Autodesk Inventor part; units mm, degrees
(part 2 of 2)
  spline S182 degree 2 poles (-123.4391, 76.8536) (-123.4391, 75.1966) (-121.7718, 73.4367) (-120.2898, 73.4367) knots 0 0 0 1 2 2 2
  spline S183 degree 2 poles (-120.2898, 73.4367) (-119.7649, 73.4367) (-118.746, 73.6734) (-118.3344, 73.8587) knots 0 0 0 1 2 2 2
  spline S184 degree 2 poles (-118.3344, 73.8587) (-117.9021, 74.0645) (-117.3052, 74.4247) (-117.1096, 74.5894) knots 0 0 0 1 2 2 2
  line L455 (-117.1096, 74.5894) -> (-117.017, 74.5894)
  line L456 (-117.017, 74.5894) -> (-117.017, 72.8398)
  spline S185 degree 2 poles (-117.017, 72.8398) (-117.2949, 72.7266) (-118.1388, 72.3972) (-118.4682, 72.3046) knots 0 0 0 1 2 2 2
  spline S186 degree 2 poles (-118.4682, 72.3046) (-118.9313, 72.1708) (-119.6929, 72.037) (-120.2692, 72.037) knots 0 0 0 1 2 2 2
  spline S187 degree 2 poles (-118.4064, 78.0783) (-118.427, 78.7267) (-118.6946, 79.6735) (-118.9519, 79.9925) knots 0 0 0 1 2 2 2
  spline S188 degree 2 poles (-118.9519, 79.9925) (-119.2297, 80.3527) (-120.1045, 80.7335) (-120.7529, 80.7335) knots 0 0 0 1 2 2 2
  spline S189 degree 2 poles (-120.7529, 80.7335) (-121.391, 80.7335) (-122.2864, 80.3527) (-122.6569, 79.9822) knots 0 0 0 1 2 2 2
  spline S190 degree 2 poles (-122.6569, 79.9822) (-123.0171, 79.6014) (-123.3876, 78.6855) (-123.4391, 78.0783) knots 0 0 0 1 2 2 2
  line L457 (-123.4391, 78.0783) -> (-118.4064, 78.0783)
  line L458 (-107.8162, 72.2532) -> (-109.7819, 72.2532)
  line L459 (-109.7819, 72.2532) -> (-112.0976, 75.8347)
  line L460 (-112.0976, 75.8347) -> (-114.475, 72.2532)
  line L461 (-114.475, 72.2532) -> (-116.2966, 72.2532)
  line L462 (-116.2966, 72.2532) -> (-112.993, 76.9771)
  line L463 (-112.993, 76.9771) -> (-116.2657, 81.7833)
  line L464 (-116.2657, 81.7833) -> (-114.3, 81.7833)
  line L465 (-114.3, 81.7833) -> (-111.9947, 78.2326)
  line L466 (-111.9947, 78.2326) -> (-109.6378, 81.7833)
  line L467 (-109.6378, 81.7833) -> (-107.8162, 81.7833)
  line L468 (-107.8162, 81.7833) -> (-111.0993, 77.08)
  line L469 (-111.0993, 77.08) -> (-107.8162, 72.2532)
  spline S191 degree 2 poles (-101.2604, 73.2617) (-101.4559, 73.1177) (-102.1146, 72.6031) (-102.4233, 72.4487) knots 0 0 0 1 2 2 2
  spline S192 degree 2 poles (-102.4233, 72.4487) (-102.8453, 72.2223) (-103.6378, 71.9856) (-104.3582, 71.9856) knots 0 0 0 1 2 2 2
  spline S193 degree 2 poles (-104.3582, 71.9856) (-104.9448, 71.9856) (-106.0049, 72.4281) (-106.4062, 72.8295) knots 0 0 0 1 2 2 2
  spline S194 degree 2 poles (-106.4062, 72.8295) (-106.787, 73.2206) (-107.2502, 74.3732) (-107.2502, 75.0113) knots 0 0 0 1 2 2 2
  spline S195 degree 2 poles (-107.2502, 75.0113) (-107.2502, 75.9993) (-106.4165, 77.399) (-105.5109, 77.8004) knots 0 0 0 1 2 2 2
  spline S196 degree 2 poles (-105.5109, 77.8004) (-104.7081, 78.1709) (-102.5263, 78.4488) (-101.2604, 78.5208) knots 0 0 0 1 2 2 2
  line L470 (-101.2604, 78.5208) -> (-101.2604, 78.8296)
  spline S197 degree 2 poles (-101.2604, 78.8296) (-101.2604, 79.3853) (-101.6, 80.0749) (-101.9088, 80.2704) knots 0 0 0 1 2 2 2
  spline S198 degree 2 poles (-101.9088, 80.2704) (-102.2175, 80.466) (-103.1026, 80.5895) (-103.576, 80.5895) knots 0 0 0 1 2 2 2
  spline S199 degree 2 poles (-103.576, 80.5895) (-104.1318, 80.5895) (-105.6344, 80.2601) (-106.3857, 79.9411) knots 0 0 0 1 2 2 2
  line L471 (-106.3857, 79.9411) -> (-106.4783, 79.9411)
  line L472 (-106.4783, 79.9411) -> (-106.4783, 81.5775)
  spline S200 degree 2 poles (-106.4783, 81.5775) (-106.0357, 81.701) (-104.3788, 82.0097) (-103.5657, 82.0097) knots 0 0 0 1 2 2 2
  spline S201 degree 2 poles (-103.5657, 82.0097) (-102.5777, 82.0097) (-101.2295, 81.701) (-100.6943, 81.2996) knots 0 0 0 1 2 2 2
  spline S202 degree 2 poles (-100.6943, 81.2996) (-100.1694, 80.9085) (-99.6549, 79.6632) (-99.6549, 78.7678) knots 0 0 0 1 2 2 2
  line L473 (-99.6549, 78.7678) -> (-99.6549, 72.2532)
  line L474 (-99.6549, 72.2532) -> (-101.2604, 72.2532)
  line L475 (-101.2604, 72.2532) -> (-101.2604, 73.2617)
  line L476 (-101.2604, 74.5997) -> (-101.2604, 77.2446)
  spline S203 degree 2 poles (-101.2604, 77.2446) (-101.8367, 77.1932) (-103.576, 77.0182) (-104.1215, 76.8536) knots 0 0 0 1 2 2 2
  spline S204 degree 2 poles (-104.1215, 76.8536) (-104.7596, 76.658) (-105.5932, 75.845) (-105.5932, 75.1245) knots 0 0 0 1 2 2 2
  spline S205 degree 2 poles (-105.5932, 75.1245) (-105.5932, 74.3012) (-104.6669, 73.4676) (-103.7818, 73.4676) knots 0 0 0 1 2 2 2
  spline S206 degree 2 poles (-103.7818, 73.4676) (-103.0306, 73.4676) (-101.7955, 74.116) (-101.2604, 74.5997) knots 0 0 0 1 2 2 2
  line L477 (-89.9189, 72.2532) -> (-91.5244, 72.2532)
  line L478 (-91.5244, 72.2532) -> (-91.5244, 77.6872)
  spline S207 degree 2 poles (-91.5244, 77.6872) (-91.5244, 78.3459) (-91.6479, 79.4779) (-91.8331, 79.8176) knots 0 0 0 1 2 2 2
  spline S208 degree 2 poles (-91.8331, 79.8176) (-92.0287, 80.1778) (-92.7285, 80.5277) (-93.3254, 80.5277) knots 0 0 0 1 2 2 2
  spline S209 degree 2 poles (-93.3254, 80.5277) (-93.9224, 80.5277) (-95.1883, 79.8896) (-95.7955, 79.375) knots 0 0 0 1 2 2 2
  line L479 (-95.7955, 79.375) -> (-95.7955, 72.2532)
  line L480 (-95.7955, 72.2532) -> (-97.401, 72.2532)
  line L481 (-97.401, 72.2532) -> (-97.401, 81.7833)
  line L482 (-97.401, 81.7833) -> (-95.7955, 81.7833)
  line L483 (-95.7955, 81.7833) -> (-95.7955, 80.7232)
  spline S210 degree 2 poles (-95.7955, 80.7232) (-95.075, 81.3716) (-93.6857, 82.0509) (-92.9035, 82.0509) knots 0 0 0 1 2 2 2
  spline S211 degree 2 poles (-92.9035, 82.0509) (-91.5038, 82.0509) (-89.9189, 80.1984) (-89.9189, 78.4385) knots 0 0 0 1 2 2 2
  line L484 (-89.9189, 78.4385) -> (-89.9189, 72.2532)
  line L485 (-77.3218, 68.7437) -> (-79.2772, 68.7437)
  spline S212 degree 2 poles (-79.2772, 68.7437) (-80.7592, 70.5036) (-82.4574, 74.4453) (-82.4574, 77.1314) knots 0 0 0 1 2 2 2
  spline S213 degree 2 poles (-82.4574, 77.1314) (-82.4574, 79.7558) (-80.7798, 83.7593) (-79.2772, 85.5192) knots 0 0 0 1 2 2 2
  line L486 (-79.2772, 85.5192) -> (-77.3218, 85.5192)
  line L487 (-77.3218, 85.5192) -> (-77.3218, 85.4369)
  spline S214 degree 2 poles (-77.3218, 85.4369) (-78.0113, 84.8091) (-79.2669, 83.183) (-79.8021, 82.1023) knots 0 0 0 1 2 2 2
  spline S215 degree 2 poles (-79.8021, 82.1023) (-80.3167, 81.0526) (-80.9548, 78.5311) (-80.9548, 77.1314) knots 0 0 0 1 2 2 2
  spline S216 degree 2 poles (-80.9548, 77.1314) (-80.9548, 75.67) (-80.3373, 73.2514) (-79.8021, 72.1605) knots 0 0 0 1 2 2 2
  spline S217 degree 2 poles (-79.8021, 72.1605) (-79.2875, 71.1108) (-77.9805, 69.4126) (-77.3218, 68.826) knots 0 0 0 1 2 2 2
  line L488 (-77.3218, 68.826) -> (-77.3218, 68.7437)
  line L489 (-68.5635, 72.2532) -> (-74.7592, 72.2532)
  line L490 (-74.7592, 72.2532) -> (-74.7592, 73.5499)
  line L491 (-74.7592, 73.5499) -> (-72.4538, 73.5499)
  line L492 (-72.4538, 73.5499) -> (-72.4538, 82.0612)
  line L493 (-72.4538, 82.0612) -> (-74.7592, 82.0612)
  line L494 (-74.7592, 82.0612) -> (-74.7592, 83.2241)
  spline S218 degree 2 poles (-74.7592, 83.2241) (-73.4521, 83.2241) (-72.2171, 83.9651) (-72.1348, 84.9943) knots 0 0 0 1 2 2 2
  line L495 (-72.1348, 84.9943) -> (-70.8174, 84.9943)
  line L496 (-70.8174, 84.9943) -> (-70.8174, 73.5499)
  line L497 (-70.8174, 73.5499) -> (-68.5635, 73.5499)
  line L498 (-68.5635, 73.5499) -> (-68.5635, 72.2532)
  line L499 (-60.9477, 85.5192) -> (-65.9186, 69.495)
  line L500 (-65.9186, 69.495) -> (-67.3594, 69.495)
  line L501 (-67.3594, 69.495) -> (-62.4091, 85.5192)
  line L502 (-62.4091, 85.5192) -> (-60.9477, 85.5192)
  spline S219 degree 2 poles (-55.7092, 71.965) (-56.656, 71.965) (-58.21, 72.531) (-58.7555, 73.0559) knots 0 0 0 1 2 2 2
  spline S220 degree 2 poles (-58.7555, 73.0559) (-59.2907, 73.5705) (-59.8464, 74.9702) (-59.8464, 75.7626) knots 0 0 0 1 2 2 2
  spline S221 degree 2 poles (-59.8464, 75.7626) (-59.8464, 76.7918) (-58.7452, 78.5208) (-57.6955, 79.0354) knots 0 0 0 1 2 2 2
  line L503 (-57.6955, 79.0354) -> (-57.6955, 79.0869)
  spline S222 degree 2 poles (-57.6955, 79.0869) (-58.632, 79.6323) (-59.5377, 80.9291) (-59.5377, 81.8965) knots 0 0 0 1 2 2 2
  spline S223 degree 2 poles (-59.5377, 81.8965) (-59.5377, 83.3271) (-57.3764, 85.2413) (-55.7092, 85.2413) knots 0 0 0 1 2 2 2
  spline S224 degree 2 poles (-55.7092, 85.2413) (-53.9801, 85.2413) (-51.8909, 83.43) (-51.8909, 82.0097) knots 0 0 0 1 2 2 2
  spline S225 degree 2 poles (-51.8909, 82.0097) (-51.8909, 81.1555) (-52.8892, 79.4882) (-53.8258, 79.0148) knots 0 0 0 1 2 2 2
  line L504 (-53.8258, 79.0148) -> (-53.8258, 78.9634)
  spline S226 degree 2 poles (-53.8258, 78.9634) (-52.7143, 78.4488) (-51.5719, 76.9668) (-51.5719, 75.7935) knots 0 0 0 1 2 2 2
  spline S227 degree 2 poles (-51.5719, 75.7935) (-51.5719, 74.1674) (-53.939, 71.965) (-55.7092, 71.965) knots 0 0 0 1 2 2 2
  spline S228 degree 2 poles (-53.3215, 75.6288) (-53.3215, 76.411) (-53.939, 77.3373) (-54.8138, 77.8107) knots 0 0 0 1 2 2 2
  spline S229 degree 2 poles (-54.8138, 77.8107) (-55.1019, 77.9754) (-56.0694, 78.3561) (-56.6766, 78.6032) knots 0 0 0 1 2 2 2
  spline S230 degree 2 poles (-56.6766, 78.6032) (-57.3764, 78.14) (-58.1277, 76.7609) (-58.1277, 75.8861) knots 0 0 0 1 2 2 2
  spline S231 degree 2 poles (-58.1277, 75.8861) (-58.1277, 74.7335) (-56.7383, 73.2309) (-55.6886, 73.2309) knots 0 0 0 1 2 2 2
  spline S232 degree 2 poles (-55.6886, 73.2309) (-54.6182, 73.2309) (-53.3215, 74.5173) (-53.3215, 75.6288) knots 0 0 0 1 2 2 2
  spline S233 degree 2 poles (-53.5582, 81.9891) (-53.5582, 82.8433) (-54.7006, 83.9857) (-55.7195, 83.9857) knots 0 0 0 1 2 2 2
  spline S234 degree 2 poles (-55.7195, 83.9857) (-56.6457, 83.9857) (-57.8293, 82.9668) (-57.8293, 82.092) knots 0 0 0 1 2 2 2
  spline S235 degree 2 poles (-57.8293, 82.092) (-57.8293, 81.4643) (-57.222, 80.5895) (-56.6148, 80.2395) knots 0 0 0 1 2 2 2
  spline S236 degree 2 poles (-56.6148, 80.2395) (-56.3575, 80.0955) (-55.2666, 79.5912) (-54.8241, 79.4471) knots 0 0 0 1 2 2 2
  spline S237 degree 2 poles (-54.8241, 79.4471) (-54.0831, 80.0131) (-53.5582, 81.2173) (-53.5582, 81.9891) knots 0 0 0 1 2 2 2
  line L505 (-48.1139, 85.5192) -> (-48.4844, 80.5792)
  line L506 (-48.4844, 80.5792) -> (-49.6062, 80.5792)
  line L507 (-49.6062, 80.5792) -> (-49.9767, 85.5192)
  line L508 (-49.9767, 85.5192) -> (-48.1139, 85.5192)
  line L509 (-44.9028, 85.5192) -> (-45.2733, 80.5792)
  line L510 (-45.2733, 80.5792) -> (-46.3951, 80.5792)
  line L511 (-46.3951, 80.5792) -> (-46.7656, 85.5192)
  line L512 (-46.7656, 85.5192) -> (-44.9028, 85.5192)
  line L513 (-39.6746, 74.682) -> (-42.0623, 69.0936)
  line L514 (-42.0623, 69.0936) -> (-43.3076, 69.0936)
  line L515 (-43.3076, 69.0936) -> (-41.805, 74.682)
  line L516 (-41.805, 74.682) -> (-39.6746, 74.682)
  line L517 (-30.5253, 72.2532) -> (-36.7209, 72.2532)
  line L518 (-36.7209, 72.2532) -> (-36.7209, 73.5499)
  line L519 (-36.7209, 73.5499) -> (-34.4156, 73.5499)
  line L520 (-34.4156, 73.5499) -> (-34.4156, 82.0612)
  line L521 (-34.4156, 82.0612) -> (-36.7209, 82.0612)
  line L522 (-36.7209, 82.0612) -> (-36.7209, 83.2241)
  spline S238 degree 2 poles (-36.7209, 83.2241) (-35.4139, 83.2241) (-34.1789, 83.9651) (-34.0965, 84.9943) knots 0 0 0 1 2 2 2
  line L523 (-34.0965, 84.9943) -> (-32.7792, 84.9943)
  line L524 (-32.7792, 84.9943) -> (-32.7792, 73.5499)
  line L525 (-32.7792, 73.5499) -> (-30.5253, 73.5499)
  line L526 (-30.5253, 73.5499) -> (-30.5253, 72.2532)
  line L527 (-22.9094, 85.5192) -> (-27.8803, 69.495)
  line L528 (-27.8803, 69.495) -> (-29.3212, 69.495)
  line L529 (-29.3212, 69.495) -> (-24.3708, 85.5192)
  line L530 (-24.3708, 85.5192) -> (-22.9094, 85.5192)
  line L531 (-13.3381, 76.6168) -> (-14.851, 76.6168)
  line L532 (-14.851, 76.6168) -> (-14.851, 72.2532)
  line L533 (-14.851, 72.2532) -> (-16.4874, 72.2532)
  line L534 (-16.4874, 72.2532) -> (-16.4874, 76.6168)
  line L535 (-16.4874, 76.6168) -> (-22.0964, 76.6168)
  line L536 (-22.0964, 76.6168) -> (-22.0964, 78.4076)
  line L537 (-22.0964, 78.4076) -> (-16.4153, 84.9532)
  line L538 (-16.4153, 84.9532) -> (-14.851, 84.9532)
  line L539 (-14.851, 84.9532) -> (-14.851, 77.9856)
  line L540 (-14.851, 77.9856) -> (-13.3381, 77.9856)
  line L541 (-13.3381, 77.9856) -> (-13.3381, 76.6168)
  line L542 (-16.4874, 77.9856) -> (-16.4874, 82.9463)
  line L543 (-16.4874, 82.9463) -> (-20.7584, 77.9856)
  line L544 (-20.7584, 77.9856) -> (-16.4874, 77.9856)
  line L545 (-10.0756, 85.5192) -> (-10.4461, 80.5792)
  line L546 (-10.4461, 80.5792) -> (-11.5679, 80.5792)
  line L547 (-11.5679, 80.5792) -> (-11.9384, 85.5192)
  line L548 (-11.9384, 85.5192) -> (-10.0756, 85.5192)
  line L549 (-6.8646, 85.5192) -> (-7.2351, 80.5792)
  line L550 (-7.2351, 80.5792) -> (-8.3569, 80.5792)
  line L551 (-8.3569, 80.5792) -> (-8.7274, 85.5192)
  line L552 (-8.7274, 85.5192) -> (-6.8646, 85.5192)
  spline S239 degree 2 poles (-0.1235, 77.1314) (-0.1235, 74.4967) (-1.8113, 70.5036) (-3.3036, 68.7437) knots 0 0 0 1 2 2 2
  line L553 (-3.3036, 68.7437) -> (-5.2591, 68.7437)
  line L554 (-5.2591, 68.7437) -> (-5.2591, 68.826)
  spline S240 degree 2 poles (-5.2591, 68.826) (-4.6004, 69.4126) (-3.2728, 71.1314) (-2.7788, 72.1605) knots 0 0 0 1 2 2 2
  spline S241 degree 2 poles (-2.7788, 72.1605) (-2.2436, 73.2617) (-1.6261, 75.7112) (-1.6261, 77.1314) knots 0 0 0 1 2 2 2
  spline S242 degree 2 poles (-1.6261, 77.1314) (-1.6261, 78.5414) (-2.2539, 81.0423) (-2.7788, 82.1023) knots 0 0 0 1 2 2 2
  spline S243 degree 2 poles (-2.7788, 82.1023) (-3.2934, 83.1624) (-4.6107, 84.8502) (-5.2591, 85.4369) knots 0 0 0 1 2 2 2
  line L555 (-5.2591, 85.4369) -> (-5.2591, 85.5192)
  line L556 (-5.2591, 85.5192) -> (-3.3036, 85.5192)
  spline S244 degree 2 poles (-3.3036, 85.5192) (-1.8216, 83.7593) (-0.1235, 79.7867) (-0.1235, 77.1314) knots 0 0 0 1 2 2 2
  line L557 (-140.4719, 56.1286) -> (-145.2781, 56.1286)
  line L558 (-145.2781, 56.1286) -> (-145.2781, 57.6724)
  line L559 (-145.2781, 57.6724) -> (-140.4719, 57.6724)
  line L560 (-140.4719, 57.6724) -> (-140.4719, 56.1286)
  spline S245 degree 2 poles (-129.4288, 51.1165) (-130.8079, 51.1165) (-132.7428, 51.6929) (-133.597, 52.1045) knots 0 0 0 1 2 2 2
  line L561 (-133.597, 52.1045) -> (-133.597, 54.2246)
  line L562 (-133.597, 54.2246) -> (-133.4735, 54.2246)
  spline S246 degree 2 poles (-133.4735, 54.2246) (-132.6399, 53.4425) (-130.5301, 52.5779) (-129.5524, 52.5779) knots 0 0 0 1 2 2 2
  spline S247 degree 2 poles (-129.5524, 52.5779) (-128.1527, 52.5779) (-126.7221, 53.7409) (-126.7221, 54.698) knots 0 0 0 1 2 2 2
  spline S248 degree 2 poles (-126.7221, 54.698) (-126.7221, 55.4596) (-127.4734, 56.4065) (-128.2865, 56.6432) knots 0 0 0 1 2 2 2
  spline S249 degree 2 poles (-128.2865, 56.6432) (-128.8731, 56.8078) (-129.8508, 57.0343) (-130.5815, 57.2195) knots 0 0 0 1 2 2 2
  spline S250 degree 2 poles (-130.5815, 57.2195) (-131.2402, 57.3945) (-132.2797, 57.9194) (-132.681, 58.3413) knots 0 0 0 1 2 2 2
  spline S251 degree 2 poles (-132.681, 58.3413) (-133.0721, 58.7633) (-133.5044, 59.8954) (-133.5044, 60.6364) knots 0 0 0 1 2 2 2
  spline S252 degree 2 poles (-133.5044, 60.6364) (-133.5044, 62.1801) (-131.0961, 64.2694) (-129.2333, 64.2694) knots 0 0 0 1 2 2 2
  spline S253 degree 2 poles (-129.2333, 64.2694) (-128.163, 64.2694) (-126.2693, 63.8474) (-125.4562, 63.446) knots 0 0 0 1 2 2 2
  line L563 (-125.4562, 63.446) -> (-125.4562, 61.4288)
  line L564 (-125.4562, 61.4288) -> (-125.5797, 61.4288)
  spline S254 degree 2 poles (-125.5797, 61.4288) (-126.187, 61.9846) (-128.0806, 62.8079) (-129.1201, 62.8079) knots 0 0 0 1 2 2 2
  spline S255 degree 2 poles (-129.1201, 62.8079) (-130.2934, 62.8079) (-131.7445, 61.7067) (-131.7445, 60.8113) knots 0 0 0 1 2 2 2
  spline S256 degree 2 poles (-131.7445, 60.8113) (-131.7445, 60.0086) (-130.8903, 59.0514) (-130.0875, 58.8353) knots 0 0 0 1 2 2 2
  spline S257 degree 2 poles (-130.0875, 58.8353) (-129.5524, 58.6912) (-127.9983, 58.3207) (-127.4837, 58.1664) knots 0 0 0 1 2 2 2
  spline S258 degree 2 poles (-127.4837, 58.1664) (-126.1767, 57.765) (-124.9622, 56.1492) (-124.9622, 54.9656) knots 0 0 0 1 2 2 2
  spline S259 degree 2 poles (-124.9622, 54.9656) (-124.9622, 54.2143) (-125.5694, 52.7735) (-126.1149, 52.2692) knots 0 0 0 1 2 2 2
  spline S260 degree 2 poles (-126.1149, 52.2692) (-126.7221, 51.7134) (-128.2659, 51.1165) (-129.4288, 51.1165) knots 0 0 0 1 2 2 2
  spline S261 degree 2 poles (-120.4853, 51.1577) (-121.7924, 51.1577) (-123.2641, 52.65) (-123.2641, 54.2658) knots 0 0 0 1 2 2 2
  line L565 (-123.2641, 54.2658) -> (-123.2641, 59.5454)
  line L566 (-123.2641, 59.5454) -> (-124.3447, 59.5454)
  line L567 (-124.3447, 59.5454) -> (-124.3447, 60.8731)
  line L568 (-124.3447, 60.8731) -> (-123.2641, 60.8731)
  line L569 (-123.2641, 60.8731) -> (-123.2641, 63.6107)
  line L570 (-123.2641, 63.6107) -> (-121.6586, 63.6107)
  line L571 (-121.6586, 63.6107) -> (-121.6586, 60.8731)
  line L572 (-121.6586, 60.8731) -> (-118.7049, 60.8731)
  line L573 (-118.7049, 60.8731) -> (-118.7049, 59.5454)
  line L574 (-118.7049, 59.5454) -> (-121.6586, 59.5454)
  line L575 (-121.6586, 59.5454) -> (-121.6586, 55.0068)
  spline S262 degree 2 poles (-121.6586, 55.0068) (-121.6586, 54.2864) (-121.6071, 53.4939) (-121.4322, 53.1543) knots 0 0 0 1 2 2 2
  spline S263 degree 2 poles (-121.4322, 53.1543) (-121.2881, 52.8558) (-120.6397, 52.5574) (-120.084, 52.5574) knots 0 0 0 1 2 2 2
  spline S264 degree 2 poles (-120.084, 52.5574) (-119.6929, 52.5574) (-118.9622, 52.7941) (-118.7975, 52.8661) knots 0 0 0 1 2 2 2
  line L576 (-118.7975, 52.8661) -> (-118.7049, 52.8661)
  line L577 (-118.7049, 52.8661) -> (-118.7049, 51.4253)
  spline S265 degree 2 poles (-118.7049, 51.4253) (-119.1577, 51.3018) (-120.084, 51.1577) (-120.4853, 51.1577) knots 0 0 0 1 2 2 2
  spline S266 degree 2 poles (-113.384, 51.1268) (-115.6688, 51.1268) (-118.18, 53.6895) (-118.18, 56.0566) knots 0 0 0 1 2 2 2
  spline S267 degree 2 poles (-118.18, 56.0566) (-118.18, 58.3825) (-115.7408, 61.1407) (-113.7751, 61.1407) knots 0 0 0 1 2 2 2
  spline S268 degree 2 poles (-113.7751, 61.1407) (-112.89, 61.1407) (-111.5212, 60.6261) (-111.0169, 60.0806) knots 0 0 0 1 2 2 2
  spline S269 degree 2 poles (-111.0169, 60.0806) (-110.5024, 59.5352) (-109.9569, 57.9605) (-109.9569, 56.8181) knots 0 0 0 1 2 2 2
  line L578 (-109.9569, 56.8181) -> (-109.9569, 55.9433)
  line L579 (-109.9569, 55.9433) -> (-116.5539, 55.9433)
  spline S270 degree 2 poles (-116.5539, 55.9433) (-116.5539, 54.2864) (-114.8866, 52.5265) (-113.4046, 52.5265) knots 0 0 0 1 2 2 2
  spline S271 degree 2 poles (-113.4046, 52.5265) (-112.8797, 52.5265) (-111.8609, 52.7632) (-111.4492, 52.9484) knots 0 0 0 1 2 2 2
  spline S272 degree 2 poles (-111.4492, 52.9484) (-111.0169, 53.1543) (-110.42, 53.5145) (-110.2245, 53.6792) knots 0 0 0 1 2 2 2
  line L580 (-110.2245, 53.6792) -> (-110.1318, 53.6792)
  line L581 (-110.1318, 53.6792) -> (-110.1318, 51.9296)
  spline S273 degree 2 poles (-110.1318, 51.9296) (-110.4097, 51.8164) (-111.2536, 51.487) (-111.583, 51.3944) knots 0 0 0 1 2 2 2
  spline S274 degree 2 poles (-111.583, 51.3944) (-112.0461, 51.2606) (-112.8077, 51.1268) (-113.384, 51.1268) knots 0 0 0 1 2 2 2
  spline S275 degree 2 poles (-111.5212, 57.1681) (-111.5418, 57.8164) (-111.8094, 58.7633) (-112.0667, 59.0823) knots 0 0 0 1 2 2 2
  spline S276 degree 2 poles (-112.0667, 59.0823) (-112.3446, 59.4425) (-113.2194, 59.8233) (-113.8677, 59.8233) knots 0 0 0 1 2 2 2
  spline S277 degree 2 poles (-113.8677, 59.8233) (-114.5058, 59.8233) (-115.4012, 59.4425) (-115.7717, 59.072) knots 0 0 0 1 2 2 2
  spline S278 degree 2 poles (-115.7717, 59.072) (-116.1319, 58.6912) (-116.5024, 57.7753) (-116.5539, 57.1681) knots 0 0 0 1 2 2 2
  line L582 (-116.5539, 57.1681) -> (-111.5212, 57.1681)
  spline S279 degree 2 poles (-104.1935, 51.1268) (-106.4783, 51.1268) (-108.9895, 53.6895) (-108.9895, 56.0566) knots 0 0 0 1 2 2 2
  spline S280 degree 2 poles (-108.9895, 56.0566) (-108.9895, 58.3825) (-106.5503, 61.1407) (-104.5846, 61.1407) knots 0 0 0 1 2 2 2
  spline S281 degree 2 poles (-104.5846, 61.1407) (-103.6995, 61.1407) (-102.3307, 60.6261) (-101.8264, 60.0806) knots 0 0 0 1 2 2 2
  spline S282 degree 2 poles (-101.8264, 60.0806) (-101.3118, 59.5352) (-100.7664, 57.9605) (-100.7664, 56.8181) knots 0 0 0 1 2 2 2
  line L583 (-100.7664, 56.8181) -> (-100.7664, 55.9433)
  line L584 (-100.7664, 55.9433) -> (-107.3634, 55.9433)
  spline S283 degree 2 poles (-107.3634, 55.9433) (-107.3634, 54.2864) (-105.6961, 52.5265) (-104.2141, 52.5265) knots 0 0 0 1 2 2 2
  spline S284 degree 2 poles (-104.2141, 52.5265) (-103.6892, 52.5265) (-102.6703, 52.7632) (-102.2587, 52.9484) knots 0 0 0 1 2 2 2
  spline S285 degree 2 poles (-102.2587, 52.9484) (-101.8264, 53.1543) (-101.2295, 53.5145) (-101.034, 53.6792) knots 0 0 0 1 2 2 2
  line L585 (-101.034, 53.6792) -> (-100.9413, 53.6792)
  line L586 (-100.9413, 53.6792) -> (-100.9413, 51.9296)
  spline S286 degree 2 poles (-100.9413, 51.9296) (-101.2192, 51.8164) (-102.0631, 51.487) (-102.3925, 51.3944) knots 0 0 0 1 2 2 2
  spline S287 degree 2 poles (-102.3925, 51.3944) (-102.8556, 51.2606) (-103.6172, 51.1268) (-104.1935, 51.1268) knots 0 0 0 1 2 2 2
  spline S288 degree 2 poles (-102.3307, 57.1681) (-102.3513, 57.8164) (-102.6189, 58.7633) (-102.8762, 59.0823) knots 0 0 0 1 2 2 2
  spline S289 degree 2 poles (-102.8762, 59.0823) (-103.1541, 59.4425) (-104.0288, 59.8233) (-104.6772, 59.8233) knots 0 0 0 1 2 2 2
  spline S290 degree 2 poles (-104.6772, 59.8233) (-105.3153, 59.8233) (-106.2107, 59.4425) (-106.5812, 59.072) knots 0 0 0 1 2 2 2
  spline S291 degree 2 poles (-106.5812, 59.072) (-106.9414, 58.6912) (-107.3119, 57.7753) (-107.3634, 57.1681) knots 0 0 0 1 2 2 2
  line L587 (-107.3634, 57.1681) -> (-102.3307, 57.1681)
  line L588 (-97.5039, 51.3429) -> (-99.1094, 51.3429)
  line L589 (-99.1094, 51.3429) -> (-99.1094, 64.609)
  line L590 (-99.1094, 64.609) -> (-97.5039, 64.609)
  line L591 (-97.5039, 64.609) -> (-97.5039, 51.3429)
  line L592 (-84.8039, 47.8335) -> (-86.7593, 47.8335)
  spline S292 degree 2 poles (-86.7593, 47.8335) (-88.2413, 49.5933) (-89.9395, 53.5351) (-89.9395, 56.2212) knots 0 0 0 1 2 2 2
  spline S293 degree 2 poles (-89.9395, 56.2212) (-89.9395, 58.8456) (-88.2619, 62.8491) (-86.7593, 64.609) knots 0 0 0 1 2 2 2
  line L593 (-86.7593, 64.609) -> (-84.8039, 64.609)
  line L594 (-84.8039, 64.609) -> (-84.8039, 64.5266)
  spline S294 degree 2 poles (-84.8039, 64.5266) (-85.4934, 63.8989) (-86.749, 62.2728) (-87.2842, 61.1921) knots 0 0 0 1 2 2 2
  spline S295 degree 2 poles (-87.2842, 61.1921) (-87.7988, 60.1424) (-88.4369, 57.6209) (-88.4369, 56.2212) knots 0 0 0 1 2 2 2
  spline S296 degree 2 poles (-88.4369, 56.2212) (-88.4369, 54.7598) (-87.8194, 52.3412) (-87.2842, 51.2503) knots 0 0 0 1 2 2 2
  spline S297 degree 2 poles (-87.2842, 51.2503) (-86.7696, 50.2006) (-85.4626, 48.5024) (-84.8039, 47.9158) knots 0 0 0 1 2 2 2
  line L595 (-84.8039, 47.9158) -> (-84.8039, 47.8335)
  spline S298 degree 2 poles (-77.6923, 52.3515) (-77.8878, 52.2074) (-78.5465, 51.6929) (-78.8553, 51.5385) knots 0 0 0 1 2 2 2
  spline S299 degree 2 poles (-78.8553, 51.5385) (-79.2772, 51.3121) (-80.0697, 51.0754) (-80.7901, 51.0754) knots 0 0 0 1 2 2 2
  spline S300 degree 2 poles (-80.7901, 51.0754) (-81.3767, 51.0754) (-82.4368, 51.5179) (-82.8382, 51.9193) knots 0 0 0 1 2 2 2
  spline S301 degree 2 poles (-82.8382, 51.9193) (-83.219, 52.3104) (-83.6821, 53.463) (-83.6821, 54.1011) knots 0 0 0 1 2 2 2
  spline S302 degree 2 poles (-83.6821, 54.1011) (-83.6821, 55.0891) (-82.8485, 56.4888) (-81.9428, 56.8902) knots 0 0 0 1 2 2 2
  spline S303 degree 2 poles (-81.9428, 56.8902) (-81.14, 57.2607) (-78.9582, 57.5386) (-77.6923, 57.6106) knots 0 0 0 1 2 2 2
  line L596 (-77.6923, 57.6106) -> (-77.6923, 57.9194)
  spline S304 degree 2 poles (-77.6923, 57.9194) (-77.6923, 58.4751) (-78.0319, 59.1647) (-78.3407, 59.3602) knots 0 0 0 1 2 2 2
  spline S305 degree 2 poles (-78.3407, 59.3602) (-78.6494, 59.5557) (-79.5345, 59.6792) (-80.0079, 59.6792) knots 0 0 0 1 2 2 2
  spline S306 degree 2 poles (-80.0079, 59.6792) (-80.5637, 59.6792) (-82.0663, 59.3499) (-82.8176, 59.0309) knots 0 0 0 1 2 2 2
  line L597 (-82.8176, 59.0309) -> (-82.9102, 59.0309)
  line L598 (-82.9102, 59.0309) -> (-82.9102, 60.6672)
  spline S307 degree 2 poles (-82.9102, 60.6672) (-82.4677, 60.7907) (-80.8107, 61.0995) (-79.9977, 61.0995) knots 0 0 0 1 2 2 2
  spline S308 degree 2 poles (-79.9977, 61.0995) (-79.0096, 61.0995) (-77.6614, 60.7907) (-77.1263, 60.3894) knots 0 0 0 1 2 2 2
  spline S309 degree 2 poles (-77.1263, 60.3894) (-76.6014, 59.9983) (-76.0868, 58.753) (-76.0868, 57.8576) knots 0 0 0 1 2 2 2
  line L599 (-76.0868, 57.8576) -> (-76.0868, 51.3429)
  line L600 (-76.0868, 51.3429) -> (-77.6923, 51.3429)
  line L601 (-77.6923, 51.3429) -> (-77.6923, 52.3515)
  line L602 (-77.6923, 53.6895) -> (-77.6923, 56.3344)
  spline S310 degree 2 poles (-77.6923, 56.3344) (-78.2686, 56.283) (-80.0079, 56.108) (-80.5534, 55.9433) knots 0 0 0 1 2 2 2
  spline S311 degree 2 poles (-80.5534, 55.9433) (-81.1915, 55.7478) (-82.0251, 54.9348) (-82.0251, 54.2143) knots 0 0 0 1 2 2 2
  spline S312 degree 2 poles (-82.0251, 54.2143) (-82.0251, 53.391) (-81.0989, 52.5574) (-80.2138, 52.5574) knots 0 0 0 1 2 2 2
  spline S313 degree 2 poles (-80.2138, 52.5574) (-79.4625, 52.5574) (-78.2275, 53.2057) (-77.6923, 53.6895) knots 0 0 0 1 2 2 2
  line L603 (-66.3508, 51.3429) -> (-67.9563, 51.3429)
  line L604 (-67.9563, 51.3429) -> (-67.9563, 56.777)
  spline S314 degree 2 poles (-67.9563, 56.777) (-67.9563, 57.4356) (-68.0798, 58.5677) (-68.2651, 58.9074) knots 0 0 0 1 2 2 2
  spline S315 degree 2 poles (-68.2651, 58.9074) (-68.4606, 59.2676) (-69.1605, 59.6175) (-69.7574, 59.6175) knots 0 0 0 1 2 2 2
  spline S316 degree 2 poles (-69.7574, 59.6175) (-70.3543, 59.6175) (-71.6202, 58.9794) (-72.2274, 58.4648) knots 0 0 0 1 2 2 2
  line L605 (-72.2274, 58.4648) -> (-72.2274, 51.3429)
  line L606 (-72.2274, 51.3429) -> (-73.8329, 51.3429)
  line L607 (-73.8329, 51.3429) -> (-73.8329, 60.8731)
  line L608 (-73.8329, 60.8731) -> (-72.2274, 60.8731)
  line L609 (-72.2274, 60.8731) -> (-72.2274, 59.813)
  spline S317 degree 2 poles (-72.2274, 59.813) (-71.507, 60.4614) (-70.1176, 61.1407) (-69.3354, 61.1407) knots 0 0 0 1 2 2 2
  spline S318 degree 2 poles (-69.3354, 61.1407) (-67.9357, 61.1407) (-66.3508, 59.2882) (-66.3508, 57.5283) knots 0 0 0 1 2 2 2
  line L610 (-66.3508, 57.5283) -> (-66.3508, 51.3429)
  line L611 (-56.6148, 60.8731) -> (-61.7401, 47.8335)
  line L612 (-61.7401, 47.8335) -> (-63.4588, 47.8335)
  line L613 (-63.4588, 47.8335) -> (-61.7504, 51.8061)
  line L614 (-61.7504, 51.8061) -> (-65.2084, 60.8731)
  line L615 (-65.2084, 60.8731) -> (-63.4794, 60.8731)
  line L616 (-63.4794, 60.8731) -> (-60.8756, 53.813)
  line L617 (-60.8756, 53.813) -> (-58.2821, 60.8731)
  line L618 (-58.2821, 60.8731) -> (-56.6148, 60.8731)
  spline S319 degree 2 poles (-50.7897, 56.2212) (-50.7897, 53.5865) (-52.4776, 49.5933) (-53.9699, 47.8335) knots 0 0 0 1 2 2 2
  line L619 (-53.9699, 47.8335) -> (-55.9253, 47.8335)
  line L620 (-55.9253, 47.8335) -> (-55.9253, 47.9158)
  spline S320 degree 2 poles (-55.9253, 47.9158) (-55.2666, 48.5024) (-53.939, 50.2211) (-53.445, 51.2503) knots 0 0 0 1 2 2 2
  spline S321 degree 2 poles (-53.445, 51.2503) (-52.9098, 52.3515) (-52.2923, 54.801) (-52.2923, 56.2212) knots 0 0 0 1 2 2 2
  spline S322 degree 2 poles (-52.2923, 56.2212) (-52.2923, 57.6312) (-52.9201, 60.1321) (-53.445, 61.1921) knots 0 0 0 1 2 2 2
  spline S323 degree 2 poles (-53.445, 61.1921) (-53.9596, 62.2522) (-55.2769, 63.94) (-55.9253, 64.5266) knots 0 0 0 1 2 2 2
  line L621 (-55.9253, 64.5266) -> (-55.9253, 64.609)
  line L622 (-55.9253, 64.609) -> (-53.9699, 64.609)
  spline S324 degree 2 poles (-53.9699, 64.609) (-52.4878, 62.8491) (-50.7897, 58.8765) (-50.7897, 56.2212) knots 0 0 0 1 2 2 2
  point P0 (0, 0)
  point P1 (0, 127)
  point P2 (0, 152.4)
  point P3 (-146.05, 0)
  point P4 (-152.4, 0)
  dimension "d4" = 25.4
  dimension "d5" = 6.35
  constraints: 4 midpoint, 1 horizontal alignment, 1 vertical alignment, 2 other
  measures "d4" distance between parallel lines of L0 L2
  measures "d5" distance between parallel lines of L1 L5
emboss "Emboss1" sketch "Sketch2" operation cut depth 0.254 direction (0, 0, -1)
fillet "Fillet1" radius 3.175 4 edges at (-152.4, 152.4, -12.7) (152.4, 152.4, -12.7) (152.4, -152.4, -12.7) (-152.4, -152.4, -12.7)
body "Solid1"
